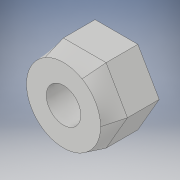
# Autodesk Inventor part: RobotArm Nut3
Saved by Autodesk Inventor 2018 (Build 220112000, 112)
## iProperties
Created: 2018-01-20
Part Number: RobotArm Nut3
Material: Generic
Document SubType Name: Modeling
Designer: lopez.xavier
Density: 1 g/cm^3
Appearance: Default
Author: lopez.xavier
Autodesk Inventor part; units mm, degrees
ref_plane "YZ Plane" through (0, 0, 0) normal (1, 0, 0) x (0, 1, 0)
ref_plane "XZ Plane" through (0, 0, 0) normal (0, 1, 0) x (-1, 0, 0)
sketch "Sketch1" plane through (0, 0, 0) normal (0, 0, 1) x (1, 0, 0)
  line L0 (2.5663, 4.445) -> (5.1326, 0)
  line L1 (5.1326, 0) -> (2.5663, -4.445)
  line L2 (2.5663, -4.445) -> (-2.5663, -4.445)
  line L3 (-2.5663, -4.445) -> (-5.1326, 0)
  line L4 (-5.1326, 0) -> (-2.5663, 4.445)
  line L5 (-2.5663, 4.445) -> (2.5663, 4.445)
  line L6 (0, 0) -> (0.7817, 0)
  dimension "d0" = 8.89
  constraints: 14 end point, 1 coincident, 1 horizontal, 1 parallel, 13 other
  measures "d0" distance between parallel lines of L5 L2
extrude "Extrusion1" add sketch "Sketch1" along normal blind 3.81
sketch "Sketch2" plane through (0, 0, 3.81) normal (0, 0, 1) x (1, 0, 0)
  line L0 (5.1326, 0) -> (2.5663, 4.445) projected
  line L1 (2.5663, 4.445) -> (-2.5663, 4.445) projected
  line L2 (-2.5663, 4.445) -> (-5.1326, 0) projected
  line L3 (-5.1326, 0) -> (-2.5663, -4.445) projected
  line L4 (-2.5663, -4.445) -> (2.5663, -4.445) projected
  line L5 (2.5663, -4.445) -> (5.1326, 0) projected
  point P0 (0, 0)
ref_plane "Work Plane1" through (0, 0, 6.35) normal (0, 0, 1) x (1, 0, 0)
sketch "Sketch3" plane through (0, 0, 6.35) normal (0, 0, 1) x (1, 0, 0)
  circle A0 centre (0, 0) radius 4.445
  dimension "d4" = 8.89
  constraints: 1 centre point, 1 coincident
  measures "d4" diameter of A0
loft "Loft1" add profiles "Sketch2", "Sketch3"
sketch "Sketch4" plane through (0, 0, 6.35) normal (0, 0, 1) x (1, 0, 0)
  circle A0 centre (0, 0) radius 2.0701
  dimension "d9" = 4.1402
  constraints: 1 centre point, 1 coincident
  measures "d9" diameter of A0
extrude "Extrusion2" cut sketch "Sketch4" against normal blind 25.4
body "Solid1"
